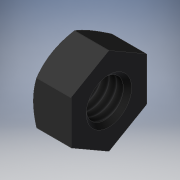
# Autodesk Inventor part: SLBNR6
Saved by Autodesk Inventor 2019 (Build 230136000, 136)
## iProperties
Created: 2024-01-23
Part Number: SLBNR6
Material: Generic
Catalog Web Link: www.cadenas.de
Description: LBNR, LBNL, SLBNR, SLBNL, KNTR, KNTL, SKNTR-Nuts
Vendor: MISUMI
Document SubType Name: Modeling
Designer: psAdmin
Manufacturer: MISUMI
Mass: 0.332096 g
Surface Area: 3.72218 cm^2
Volume: 0.332096 cm^3
Density: 1 g/cm^3
Appearance: PSOLRGB-175-175-175
Category: PARTsolutions
Company: MISUMI
Title: SLBNR6
Author: Cadenas PARTsolutions
Comments: Nuts
PSOL_IDENT_0: {$CADENAS_DATA/23d-libs/misumi/metric/27_screws_nuts/slbnl.prj},199 {VTYP=3D},{NB=SLBNR6},{LINA=SLBN
PSOL_IDENT_1: R6},{NN=LBNR, LBNL, SLBNR, SLBNL, KNTR, KNTL, SKNTR},{DATE=03.06.2021 03:35:45},{GEOMDATE=05.11.2010
PSOL_IDENT_2: 00:00:00},{VERSION=},{LINEID=50},{WBVAR=TRS,MAT,CS},{WBNUMERIC=}  {NB=SLBNR6},{LINA=SLBNR6},{KT=DUM
PSOL_IDENT_3: MY},{PN=SLBNR6},{TS=LBN},{TRS=R},{MAT=S},{ST=-},{CS=1},{M1=6},{M=6.0},{P=1.00},{B=10.0},{EE=11.5},{T=
PSOL_IDENT_4: 5.0},{T1=0.0},{TFX=5.0},{T1FX=3.6},{CALG='1','JIS Class 1','2','JIS Class 3'},{TRSALG= 'R', 'Right-H
PSOL_IDENT_5: and Thread', 'L', 'Left-Hand Thread' },{MATALG= '', 'SWCH Carbon Steel', 'S', '304 Stainless Steel'
PSOL_IDENT_6: }
NB: SLBNR6
NN: LBNR, LBNL, SLBNR, SLBNL, KNTR, KNTL, SKNTR
NT: Nuts
NBSYN: $PN.
LINA: SLBNR6
CATALOG: Misumi
PN: SLBNR6
TRS: Right-Hand Thread
MAT: 304 Stainless Steel Equivalent
ST: -
CS: JIS Class 1
M1: 6
P: 1
B: 10
EE: 11.5
T: 5
T1: 0
SUPPLIER: MISUMI
ARTICLENO: SLBNR6
BOMINFO: SLBNR6
CREATOR: CADENAS GmbH
Autodesk Inventor part; units mm, degrees
sketch "Sketch_1" plane through (0, 0, 0) normal (0, 0, 1) x (1, 0, 0)
  line L0 (2.5, 0) -> (-2.5, 0)
  line L1 (-2.5, 0) -> (-2.5, 5)
  line L2 (-2.5, 5) -> (-2.067, 5.75)
  line L3 (-2.067, 5.75) -> (2.5, 5.75)
  line L4 (2.5, 5.75) -> (2.5, 0)
  line L5 (2.5, 0) -> (-2.5, 0)
  constraints: 12 end point
revolve "Revolution1" add sketch "Sketch_1" angle 360 about axis through (2.5, 0, 0) along (1, 0, 0)
sketch "Sketch_2" plane through (0, 0, 0) normal (0, 0, 1) x (1, 0, 0)
  line L0 (2.5, 0) -> (-2.5, 0)
  line L1 (-2.5, 0) -> (-2.5, 3)
  line L2 (-2.5, 3) -> (-1.9585, 2.4585)
  line L3 (-1.9585, 2.4585) -> (1.9585, 2.4585)
  line L4 (1.9585, 2.4585) -> (2.5, 3)
  line L5 (2.5, 3) -> (2.5, 0)
  line L6 (2.5, 0) -> (-2.5, 0)
  constraints: 14 end point
revolve "Revolution2" cut sketch "Sketch_2" angle 360 about axis through (2.5, 0, 0) along (1, 0, 0)
thread "Thread1" size "M6x1" class "6H" standard "ISO Metric profile" full length
sketch "Sketch_3" plane through (0, 0, 0) normal (1, 0, 0) x (0, 1, 0)
  line L0 (-10, 10) -> (-10, -10)
  line L1 (-10, -10) -> (10, -10)
  line L2 (10, -10) -> (10, 10)
  line L3 (10, 10) -> (-10, 10)
  line L4 (-2.8868, 5) -> (-5.7735, 0)
  line L5 (-5.7735, 0) -> (-2.8868, -5)
  line L6 (-2.8868, -5) -> (2.8868, -5)
  line L7 (2.8868, -5) -> (5.7735, 0)
  line L8 (5.7735, 0) -> (2.8868, 5)
  line L9 (2.8868, 5) -> (-2.8868, 5)
  constraints: 20 end point
extrude "Extrusion1" cut sketch "Sketch_3" along normal mid plane 5
ref_plane "cp_XY" through (2.5, 0, 0) normal (1, 0, 0) x (0, 0, -1)
ref_plane "cp_YZ" through (2.5, 0, 0) normal (0, 0, -1) x (0, 1, 0)
ref_plane "cp_ZX" through (2.5, 0, 0) normal (0, 1, 0) x (1, 0, 0)
ref_plane "nut_to_screw_XY" through (0, 0, 0) normal (1, 0, 0) x (0, 0, -1)
ref_plane "nut_to_screw_YZ" through (0, 0, 0) normal (0, 0, -1) x (0, 1, 0)
ref_plane "nut_to_screw_ZX" through (0, 0, 0) normal (0, 1, 0) x (1, 0, 0)
body "Solid1"
